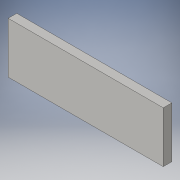
# Autodesk Inventor part: Aidasn Sherry Breadboard
Saved by Autodesk Inventor 2016 (Build 200138000, 138)
## iProperties
Created: 2016-10-11
Part Number: Aidasn Sherry Breadboard
Material: Generic
Document SubType Name: Modeling
Designer: sherra
Density: 1 g/cm^3
Appearance: Default
Author: sherra
Autodesk Inventor part; units mm, degrees
ref_plane "YZ Plane" through (0, 0, 0) normal (1, 0, 0) x (0, 1, 0)
ref_plane "XZ Plane" through (0, 0, 0) normal (0, 1, 0) x (-1, 0, 0)
ref_plane "XY Plane" through (0, 0, 0) normal (0, 0, 1) x (1, 0, 0)
sketch "Sketch1" plane through (0, 0, 0) normal (0, 0, 1) x (1, 0, 0)
  line L0 (-72.5336, 22.8993) -> (92.5664, 22.8993)
  line L1 (92.5664, 22.8993) -> (92.5664, -31.3805)
  line L2 (92.5664, -31.3805) -> (-72.5336, -31.3805)
  line L3 (-72.5336, -31.3805) -> (-72.5336, 22.8993)
  point P0 (0, 0)
  dimension "d0" = 54.2798
  dimension "d1" = 165.1
  constraints: 8 end point, 2 parallel, 1 horizontal, 1 perpendicular
  measures "d0" distance of L0.end L1.end
  measures "d1" distance of L0.start L0.end
extrude "Extrusion1" add sketch "Sketch1" along normal blind 9.144
body "Solid1"
